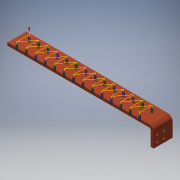
# Autodesk Inventor part: 17-0028-0017
Saved by Autodesk Inventor 2016 SP2 (Build 200236200, 236)
## iProperties
Category: IOP
Company: Universiteit van Amsterdam
BeforeDocSave0: Open Form
Created: 2017-11-01
Part Number: 17-0028-0017
Material: Copper
Document SubType Name: Modeling
Designer: Daan Giesen
Density: 8.94 g/cm^3
Appearance: Copper - Satin
Mass: 704.361 g
Surface Area: 341.431 cm^2
Volume: 78.7876 cm^3
Project: Digital PID Loop
Cost Center: 17-0028
User Status: CNC
Authority: Reichsöllner, Lukas
Description: Upper bus bar
Author: Daan Giesen
Title: Digital PID Loop
Revision Number: A.1
Autodesk Inventor part; units mm, degrees
ref_plane "YZ Plane" through (0, 0, 0) normal (1, 0, 0) x (0, 1, 0)
ref_plane "XZ Plane" through (0, 0, 0) normal (0, 1, 0) x (-1, 0, 0)
ref_plane "XY Plane" through (0, 0, 0) normal (0, 0, 1) x (1, 0, 0)
sketch "Sketch1" plane through (0, 0, 0) normal (0, 0, 1) x (1, 0, 0)
  line L0 (0, 28) -> (0, -28) construction
  line L1 (-368.1504, 0) -> (64.8584, 0) construction
  line L2 (-3, -20) -> (3, -20)
  line L3 (3, -20) -> (3, 20)
  line L4 (3, 20) -> (-3, 20)
  line L5 (-3, 20) -> (-3, -20)
  line L6 (-3, -20) -> (3, 20) construction
  line L7 (3, -20) -> (-3, 20) construction
  point P0 (0, 0)
  dimension "d0" = 40
  dimension "d1" = 6
  constraints: 12 end point, 2 midpoint, 2 parallel, 1 horizontal, 1 perpendicular
  measures "d0" distance of L2.end L3.end
  measures "d1" distance of L3.end L4.end
extrude "Extrusion1" add sketch "Sketch1" along normal blind 345
sketch "Sketch2" plane through (3, -20, 0) normal (1, 0, 0) x (0, 0, -1)
  line L0 (0, 0) -> (0, 40) projected
  line L1 (0, 40) -> (-345, 40) projected
  line L2 (-345, 0) -> (-345, 40) projected
  line L3 (0, 0) -> (-345, 0) projected
  line L4 (-30, 0) -> (-30, 40)
  point P0 (0, 20)
  dimension "d4" = 315
  constraints: 2 end point, 2 point on line, 1 perpendicular
  measures "d4" distance between parallel lines of L2 L4
bend part "Bend Part1" radius 10 angle 90 line through (3, -20, 30) along (0, 1, 0) centre toward (-1, 0, 0) moving side (0, 0, 1) both sides no
sketch "Sketch4" plane through (-306.292, 20, 40) normal (0, 0, 1) x (1, 0, 0)
  arc A0 (269.6, -17.361) -> (273.1, -17.361) centre (271.35, -17.361) ccw projected
  arc A1 (256.6, -17.361) -> (260.1, -17.361) centre (258.35, -17.361) ccw projected
  arc A2 (243.6, -17.361) -> (247.1, -17.361) centre (245.35, -17.361) ccw projected
  arc A3 (230.6, -17.361) -> (234.1, -17.361) centre (232.35, -17.361) ccw projected
  arc A4 (217.6, -17.361) -> (221.1, -17.361) centre (219.35, -17.361) ccw projected
  arc A5 (204.6, -17.361) -> (208.1, -17.361) centre (206.35, -17.361) ccw projected
  arc A6 (191.6, -17.361) -> (195.1, -17.361) centre (193.35, -17.361) ccw projected
  arc A7 (178.6, -17.361) -> (182.1, -17.361) centre (180.35, -17.361) ccw projected
  arc A8 (165.6, -17.361) -> (169.1, -17.361) centre (167.35, -17.361) ccw projected
  arc A9 (152.6, -17.361) -> (156.1, -17.361) centre (154.35, -17.361) ccw projected
  line L0 (139.35, -15.071) -> (139.35, -21.931) projected
  line L1 (128.75, -15.071) -> (139.35, -15.071) projected
  line L2 (128.75, -21.931) -> (128.75, -15.071) projected
  line L3 (130.62, -21.931) -> (128.75, -21.931) projected
  line L4 (130.62, -27.261) -> (130.62, -21.931) projected
  line L5 (137.48, -27.261) -> (130.62, -27.261) projected
  line L6 (137.48, -21.931) -> (137.48, -27.261) projected
  line L7 (139.35, -21.931) -> (137.48, -21.931) projected
  arc A10 (135.8, -17.361) -> (132.3, -17.361) centre (134.05, -17.361) ccw projected
  arc A11 (132.3, -17.361) -> (135.8, -17.361) centre (134.05, -17.361) ccw projected
  arc A12 (106.3, -17.361) -> (109.8, -17.361) centre (108.05, -17.361) ccw projected
  arc A13 (93.3, -17.361) -> (96.8, -17.361) centre (95.05, -17.361) ccw projected
  arc A14 (80.3, -17.361) -> (83.8, -17.361) centre (82.05, -17.361) ccw projected
  arc A15 (67.3, -17.361) -> (70.8, -17.361) centre (69.05, -17.361) ccw projected
  arc A16 (54.3, -17.361) -> (57.8, -17.361) centre (56.05, -17.361) ccw projected
  arc A17 (41.3, -17.361) -> (44.8, -17.361) centre (43.05, -17.361) ccw projected
  arc A18 (28.3, -17.361) -> (31.8, -17.361) centre (30.05, -17.361) ccw projected
  arc A19 (15.3, -17.361) -> (18.8, -17.361) centre (17.05, -17.361) ccw projected
  arc A20 (119.3, -17.361) -> (122.8, -17.361) centre (121.05, -17.361) ccw projected
  point P0 (306.292, -20)
  constraints: 20 coincident
hole "Hole2" at (-289.242, 2.639, 40) at (-276.242, 2.639, 40) at (-263.242, 2.639, 40) at (-250.242, 2.639, 40) at (-237.242, 2.639, 40) at (-224.242, 2.639, 40) at (-211.242, 2.639, 40) at (-198.242, 2.639, 40) at (-185.242, 2.639, 40) at (-172.242, 2.639, 40) at (-151.942, 2.639, 40) at (-138.942, 2.639, 40) at (-125.942, 2.639, 40) at (-112.942, 2.639, 40) at (-99.942, 2.639, 40) at (-86.942, 2.639, 40) at (-73.942, 2.639, 40) at (-60.942, 2.639, 40) at (-47.942, 2.639, 40) at (-34.942, 2.639, 40) direction (0, 0, -1) diameter 3.2 end through all
sketch "Sketch5" plane through (-306.292, 20, 40) normal (0, 0, 1) x (1, 0, 0)
  line L0 (284, -75) -> (284, 0) projected
  line L1 (299.292, 0) -> (0, 0) projected
  line L2 (299.292, -40) -> (0, -40) projected
  point P0 (306.292, -20)
  point P1 (274, -8)
  point P2 (274, -34)
  dimension "d23" = 10
  dimension "d24" = 8
  dimension "d25" = 6
  constraints: 1 vertical alignment
  measures "d23" distance from line of L0 point (274, -8)
  measures "d24" distance from line of point (274, -8) L1
  measures "d25" distance from line of point (274, -34) L2
hole "Hole3" at (-32.292, 12, 40) at (-32.292, -14, 40) direction (0, 0, -1) diameter 3.242 end through all thread size "M4x0.7" class "6H" standard "ISO Metric profile"
pattern_linear "Rectangular Pattern1" count 14 spacing 20 along (-1, 0, 0) of "Hole3"
sketch "Sketch6" plane through (-3, -20, 30) normal (-1, 0, 0) x (0, 0, 1)
  line L0 (-30, 0) -> (0, 0) projected
  line L1 (-30, 40) -> (-30, 0) projected
  line L2 (-8, 8) -> (-22, 8) construction
  line L3 (-22, 8) -> (-22, 22) construction
  line L4 (-22, 22) -> (-8, 22) construction
  line L5 (-8, 22) -> (-8, 8) construction
  line L6 (-8, 8) -> (-22, 22) construction
  line L7 (-22, 8) -> (-8, 22) construction
  point P0 (-30, 20)
  point P1 (-15, 15)
  dimension "d51" = 14
  dimension "d52" = 14
  dimension "d53" = 15
  dimension "d54" = 15
  constraints: 12 end point, 3 coincident, 2 midpoint, 2 parallel, 1 horizontal, 1 perpendicular
  measures "d51" distance of L2.end L3.end
  measures "d52" distance of L3.end L4.end
  measures "d53" distance from line of L0 point (-15, 15)
  measures "d54" distance from line of L1 point (-15, 15)
hole "Hole6" at (-3, -12, 8) at (-3, -12, 22) at (-3, 2, 22) at (-3, 2, 8) direction (1, 0, 0) diameter 5.3 end through all
body "Solid1"
